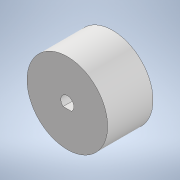
# Autodesk Inventor part: koło
Saved by Autodesk Inventor 2022.3 (Build 263350000, 350)
## iProperties
Created: 2022-12-13
Part Number: koło
Material: Generic
Document SubType Name: Modeling
Designer: komputer
Density: 1 g/cm^3
Appearance: Default
Author: komputer
Autodesk Inventor part; units mm, degrees
ref_plane "YZ Plane" through (0, 0, 0) normal (1, 0, 0) x (0, 1, 0)
ref_plane "XZ Plane" through (0, 0, 0) normal (0, 1, 0) x (-1, 0, 0)
ref_plane "XY Plane" through (0, 0, 0) normal (0, 0, 1) x (1, 0, 0)
sketch "Sketch1" plane through (0, 0, 0) normal (0, 0, 1) x (1, 0, 0)
  arc A0 (-0.4247, 0.01) -> (-2.6608, 0.01) centre (-1.5427, 1.01) ccw
  arc A1 (-2.6608, 0.01) -> (-0.4247, 0.01) centre (-1.5427, 1.01) ccw
  line L0 (-10.5427, 12.35) -> (-10.5427, -2.95)
  line L1 (-7.5427, -2.95) -> (-10.5427, -2.95)
  line L2 (-7.5427, 12.35) -> (-7.5427, -2.95)
  line L3 (-7.5427, 12.35) -> (-10.5427, 12.35)
  line L4 (-10.5427, 47.05) -> (-10.5427, 12.35)
  line L5 (-10.5427, 12.35) -> (-4.5427, 12.35)
  line L6 (-4.5427, 47.05) -> (-4.5427, 12.35)
  line L7 (-10.5427, 47.05) -> (-4.5427, 47.05)
  line L8 (1.9573, 15.05) -> (-0.8499, 15.05)
  arc A2 (-2.2355, 15.05) -> (-0.8499, 15.05) centre (-1.5427, 13.95) ccw
  line L9 (-2.2355, 15.05) -> (-5.0427, 15.05)
  arc A3 (-5.0427, 15.05) -> (-5.5427, 14.55) centre (-5.0427, 14.55) ccw
  line L10 (-5.5427, 14.55) -> (-5.5427, 12.85)
  line L11 (-5.5427, 12.85) -> (-7.0427, 12.85)
  arc A4 (-7.0427, 12.85) -> (-7.5427, 12.35) centre (-7.0427, 12.35) ccw
  line L12 (-7.5427, 12.35) -> (-7.5427, -2.45)
  arc A5 (-7.5427, -2.45) -> (-7.0427, -2.95) centre (-7.0427, -2.45) ccw
  line L13 (-7.0427, -2.95) -> (3.9573, -2.95)
  arc A6 (3.9573, -2.95) -> (4.4573, -2.45) centre (3.9573, -2.45) ccw
  line L14 (4.4573, -2.45) -> (4.4573, 12.35)
  arc A7 (4.4573, 12.35) -> (3.9573, 12.85) centre (3.9573, 12.35) ccw
  line L15 (3.9573, 12.85) -> (2.4573, 12.85)
  line L16 (2.4573, 12.85) -> (2.4573, 14.55)
  arc A8 (2.4573, 14.55) -> (1.9573, 15.05) centre (1.9573, 14.55) ccw
  circle A9 centre (-1.5427, 1.01) radius 2
  circle A10 centre (1.2073, 9.85) radius 0.45
  circle A11 centre (0.0302, 6.6603) radius 0.45
  circle A12 centre (-1.5427, 4.59) radius 0.45
  circle A13 centre (2.7073, -1.24) radius 1.25
  circle A14 centre (-5.7927, -1.24) radius 1.25
  line L17 (-1.5427, 1.01) -> (-10.5427, 1.01)
  line L18 (-10.5427, 1.01) -> (-12.5427, 1.01)
  line L19 (-12.5427, 1.01) -> (-9.5427, 1.01)
  circle A15 centre (-1.5427, 1.01) radius 8
  line L20 (-1.5427, 1.01) -> (-1.5427, -6.99)
  line L21 (-1.5427, -6.99) -> (-1.5427, -9.99)
  line L22 (-2.3734, 0.01) -> (-0.7121, 0.01)
  arc A16 (-0.7121, 0.01) -> (-2.3734, 0.01) centre (-1.5427, 1.01) ccw
  point P0 (0, 0)
extrude "Extrusion1" add sketch "Sketch1" against normal blind 9 contours A1 L20 L22 A16 L17 A0 | A0 L17 A9 L20 A1 | L17 A16 L22 L20 A1 A0 | A0 A1 L20 A9 L17 | L17 L2 A15 L14 A6 L13 L20 A9 | A9 L20 L13 A5 L2 L17 | L17 A15 L2 | L2 L1 A15 L17 | L20 A15 L1 L2 A5 L13 | L13 A6 L14 A15 L20 | A11 | A12 | A13 | A14
body "Solid1"
